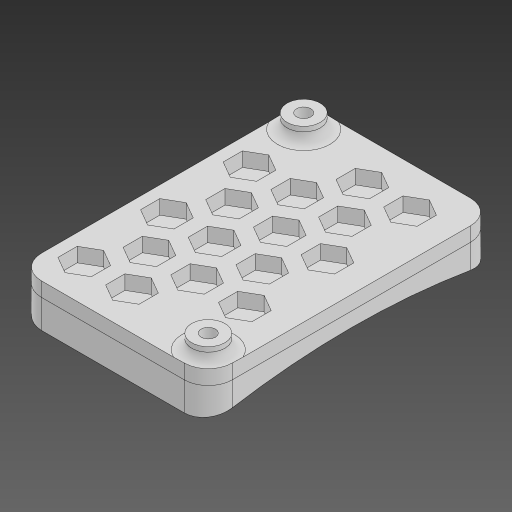
# Autodesk Inventor part: Base
Saved by Autodesk Inventor 2023.2 (Build 272271000, 271)
## iProperties
Created: 2023-04-07
Part Number: Base
Material: Generic
Document SubType Name: Modeling
Designer: jcgg2
Density: 1 g/cm^3
Appearance: Default
Mass: 14.6819 g
Surface Area: 110.672 cm^2
Volume: 14.6819 cm^3
Author: jcgg2
Autodesk Inventor part; units mm, degrees
ref_plane "YZ Plane" through (0, 0, 0) normal (1, 0, 0) x (0, 1, 0)
ref_plane "XZ Plane" through (0, 0, 0) normal (0, 1, 0) x (-1, 0, 0)
ref_plane "XY Plane" through (0, 0, 0) normal (0, 0, 1) x (1, 0, 0)
sketch "Sketch1" plane through (0, 0, 0) normal (0, 1, 0) x (-1, 0, 0)
  line L0 (-20, 30) -> (20, 30) construction
  line L1 (20, 30) -> (20, -30) construction
  line L2 (20, -30) -> (-20, -30) construction
  line L3 (-20, -30) -> (-20, 30) construction
  line L4 (-20, 30) -> (20, -30) construction
  line L5 (20, 30) -> (-20, -30) construction
  line L6 (-20, 30) -> (20, 30)
  line L7 (20, 30) -> (20, -30)
  line L8 (20, -30) -> (-20, -30)
  line L9 (-20, -30) -> (-20, 30)
  line L10 (-20, 30) -> (20, -30) construction
  line L11 (20, 30) -> (-20, -30) construction
  point P0 (0, 0)
  point P1 (-15, 25)
  point P2 (15, -25)
  dimension "d0" = 60
  dimension "d1" = 40
  dimension "d2" = 5
  dimension "d3" = 5
  dimension "d4" = 5
  dimension "d5" = 5
  constraints: 24 end point, 4 midpoint, 4 parallel, 2 horizontal, 2 perpendicular
  measures "d0" distance of L0.end L1.end
  measures "d1" distance of L1.end L2.end
  measures "d2" distance from line of L0 point (-15, 25)
  measures "d3" distance from line of L3 point (-15, 25)
  measures "d4" distance from line of L2 point (15, -25)
  measures "d5" distance from line of L1 point (15, -25)
extrude "Extrusion1" add sketch "Sketch1" along normal blind 3
hole "Hole1" at (15, 0, 25) at (-15, 0, -25) direction (0, 1, 0) diameter 3 depth 12 tip angle 118
sketch "Sketch2" plane through (0, 3, 0) normal (0, 1, 0) x (1, 0, 0)
  circle A0 centre (15, -25) radius 1.5 projected
  circle A1 centre (-15, 25) radius 1.5 projected
  line L0 (20, 30) -> (-20, 30) projected
  line L1 (-20, 30) -> (-20, -30) projected
  line L2 (-20, -30) -> (20, -30) projected
  line L3 (20, -30) -> (20, 30) projected
  circle A2 centre (15, -25) radius 3.5
  circle A3 centre (-15, 25) radius 3.5
  point P0 (0, 0)
  dimension "d15" = 2
  dimension "d16" = 2
  constraints: 2 centre point
  measures "d15" radial gap between concentric circles of A0 A2
  measures "d16" radial gap between concentric circles of A1 A3
extrude "Extrusion2" add sketch "Sketch2" along normal blind 3 contours A2 | A3
fillet "Fillet1" radius 2 2 edges at (11.5, 3, 25) (-18.5, 3, -25)
fillet "Fillet2" radius 5 4 edges at (20, 1.5, 30) (-20, 1.5, 30) (20, 1.5, -30) (-20, 1.5, -30)
sketch "Sketch3" plane through (20, 0, 25) normal (1, 0, 0) x (0, 0, -1)
  line L0 (-5, 3.0635) -> (-5, 0) projected
  line L1 (55, 0) -> (55, 3) projected
  line L2 (0, 0) -> (50, 0) projected
  line L3 (0, 0) -> (-5, 0) projected
  line L4 (55, 0) -> (50, 0) projected
  line L5 (0, 0) -> (-5, 0) projected
  line L6 (-5, 0) -> (55, 0)
  line L7 (55, 0) -> (55, -6)
  line L8 (55, -6) -> (-5, -6)
  line L9 (-5, -6) -> (-5, 0)
  line L10 (-5, 0) -> (55, 0)
  line L11 (55, 0) -> (55, -3)
  line L12 (55, -3) -> (-5, -3)
  line L13 (-5, -3) -> (-5, 0)
  arc A0 (55, -6) -> (-5, -6) centre (25, -154.5) ccw
  point P0 (25, 0)
  dimension "d21" = 6
  dimension "d22" = 3
  constraints: 16 end point, 4 parallel, 2 horizontal, 2 perpendicular, 2 point on circle, 1 centre point, 1 collinear, 1 midpoint, 1 tangent
  measures "d21" distance of L6.end L7.end
  measures "d22" distance of L10.end L11.end
extrude "Extrusion3" add sketch "Sketch3" against normal blind 40 separate body contours L2 L4 L7 L12 L9 L3 | L12 A0 L9 | L7 A0 L12
fillet "Fillet3" radius 5 4 edges at (20, -3, -30) (-20, -3, -30) (20, -3, 30) (-20, -3, 30)
sketch "Sketch4" plane through (20, 0, 25) normal (0, 1, 0) x (1, 0, 0)
  circle A0 centre (-5, 0) radius 1.5 projected
  circle A1 centre (-35, 50) radius 1.5 projected
  point P0 (-20, 25)
extrude "Extrusion4" cut sketch "Sketch4" against normal blind 40 bodies 2
sketch "Sketch5" plane through (0, 3, 0) normal (0, 1, 0) x (1, 0, 0)
  line L0 (-14, -17.9585) -> (-10.5, -19.9793)
  line L1 (-10.5, -19.9793) -> (-10.5, -24.0207)
  line L2 (-10.5, -24.0207) -> (-14, -26.0415)
  line L3 (-14, -26.0415) -> (-17.5, -24.0207)
  line L4 (-17.5, -24.0207) -> (-17.5, -19.9793)
  line L5 (-17.5, -19.9793) -> (-14, -17.9585)
  line L6 (-20, 22.7087) -> (-20, -25) projected
  line L7 (-15, -30) -> (12.7087, -30) projected
  line L8 (-14, -22) -> (-7.0718, -10) construction
  line L9 (-14, -22) -> (-7.0718, -22) construction
  line L10 (-4, -17.9585) -> (-0.5, -19.9793)
  line L11 (-0.5, -19.9793) -> (-0.5, -24.0207)
  line L12 (-0.5, -24.0207) -> (-4, -26.0415)
  line L13 (-4, -26.0415) -> (-7.5, -24.0207)
  line L14 (-7.5, -24.0207) -> (-7.5, -19.9793)
  line L15 (-7.5, -19.9793) -> (-4, -17.9585)
  line L16 (6, -17.9585) -> (9.5, -19.9793)
  line L17 (9.5, -19.9793) -> (9.5, -24.0207)
  line L18 (9.5, -24.0207) -> (6, -26.0415)
  line L19 (6, -26.0415) -> (2.5, -24.0207)
  line L20 (2.5, -24.0207) -> (2.5, -19.9793)
  line L21 (2.5, -19.9793) -> (6, -17.9585)
  line L22 (16, -17.9585) -> (19.5, -19.9793)
  line L23 (19.5, -19.9793) -> (19.5, -24.0207)
  line L24 (19.5, -24.0207) -> (16, -26.0415)
  line L25 (16, -26.0415) -> (12.5, -24.0207)
  line L26 (12.5, -24.0207) -> (12.5, -19.9793)
  line L27 (12.5, -19.9793) -> (16, -17.9585)
  line L28 (26, -17.9585) -> (29.5, -19.9793)
  line L29 (29.5, -19.9793) -> (29.5, -24.0207)
  line L30 (29.5, -24.0207) -> (26, -26.0415)
  line L31 (26, -26.0415) -> (22.5, -24.0207)
  line L32 (22.5, -24.0207) -> (22.5, -19.9793)
  line L33 (22.5, -19.9793) -> (26, -17.9585)
  line L34 (-9, -9.2983) -> (-5.5, -11.319)
  line L35 (-5.5, -11.319) -> (-5.5, -15.3605)
  line L36 (-5.5, -15.3605) -> (-9, -17.3812)
  line L37 (-9, -17.3812) -> (-12.5, -15.3605)
  line L38 (-12.5, -15.3605) -> (-12.5, -11.319)
  line L39 (-12.5, -11.319) -> (-9, -9.2983)
  line L40 (1, -9.2983) -> (4.5, -11.319)
  line L41 (4.5, -11.319) -> (4.5, -15.3605)
  line L42 (4.5, -15.3605) -> (1, -17.3812)
  line L43 (1, -17.3812) -> (-2.5, -15.3605)
  line L44 (-2.5, -15.3605) -> (-2.5, -11.319)
  line L45 (-2.5, -11.319) -> (1, -9.2983)
  line L46 (11, -9.2983) -> (14.5, -11.319)
  line L47 (14.5, -11.319) -> (14.5, -15.3605)
  line L48 (14.5, -15.3605) -> (11, -17.3812)
  line L49 (11, -17.3812) -> (7.5, -15.3605)
  line L50 (7.5, -15.3605) -> (7.5, -11.319)
  line L51 (7.5, -11.319) -> (11, -9.2983)
  line L52 (21, -9.2983) -> (24.5, -11.319)
  line L53 (24.5, -11.319) -> (24.5, -15.3605)
  line L54 (24.5, -15.3605) -> (21, -17.3812)
  line L55 (21, -17.3812) -> (17.5, -15.3605)
  line L56 (17.5, -15.3605) -> (17.5, -11.319)
  line L57 (17.5, -11.319) -> (21, -9.2983)
  line L58 (31, -9.2983) -> (34.5, -11.319)
  line L59 (34.5, -11.319) -> (34.5, -15.3605)
  line L60 (34.5, -15.3605) -> (31, -17.3812)
  line L61 (31, -17.3812) -> (27.5, -15.3605)
  line L62 (27.5, -15.3605) -> (27.5, -11.319)
  line L63 (27.5, -11.319) -> (31, -9.2983)
  line L64 (-4, -0.638) -> (-0.5, -2.6588)
  line L65 (-0.5, -2.6588) -> (-0.5, -6.7002)
  line L66 (-0.5, -6.7002) -> (-4, -8.7209)
  line L67 (-4, -8.7209) -> (-7.5, -6.7002)
  line L68 (-7.5, -6.7002) -> (-7.5, -2.6588)
  line L69 (-7.5, -2.6588) -> (-4, -0.638)
  line L70 (6, -0.638) -> (9.5, -2.6588)
  line L71 (9.5, -2.6588) -> (9.5, -6.7002)
  line L72 (9.5, -6.7002) -> (6, -8.7209)
  line L73 (6, -8.7209) -> (2.5, -6.7002)
  line L74 (2.5, -6.7002) -> (2.5, -2.6588)
  line L75 (2.5, -2.6588) -> (6, -0.638)
  line L76 (16, -0.638) -> (19.5, -2.6588)
  line L77 (19.5, -2.6588) -> (19.5, -6.7002)
  line L78 (19.5, -6.7002) -> (16, -8.7209)
  line L79 (16, -8.7209) -> (12.5, -6.7002)
  line L80 (12.5, -6.7002) -> (12.5, -2.6588)
  line L81 (12.5, -2.6588) -> (16, -0.638)
  line L82 (26, -0.638) -> (29.5, -2.6588)
  line L83 (29.5, -2.6588) -> (29.5, -6.7002)
  line L84 (29.5, -6.7002) -> (26, -8.7209)
  line L85 (26, -8.7209) -> (22.5, -6.7002)
  line L86 (22.5, -6.7002) -> (22.5, -2.6588)
  line L87 (22.5, -2.6588) -> (26, -0.638)
  line L88 (36, -0.638) -> (39.5, -2.6588)
  line L89 (39.5, -2.6588) -> (39.5, -6.7002)
  line L90 (39.5, -6.7002) -> (36, -8.7209)
  line L91 (36, -8.7209) -> (32.5, -6.7002)
  line L92 (32.5, -6.7002) -> (32.5, -2.6588)
  line L93 (32.5, -2.6588) -> (36, -0.638)
  line L94 (1, 8.0222) -> (4.5, 6.0015)
  line L95 (4.5, 6.0015) -> (4.5, 1.96)
  line L96 (4.5, 1.96) -> (1, -0.0607)
  line L97 (1, -0.0607) -> (-2.5, 1.96)
  line L98 (-2.5, 1.96) -> (-2.5, 6.0015)
  line L99 (-2.5, 6.0015) -> (1, 8.0222)
  line L100 (11, 8.0222) -> (14.5, 6.0015)
  line L101 (14.5, 6.0015) -> (14.5, 1.96)
  line L102 (14.5, 1.96) -> (11, -0.0607)
  line L103 (11, -0.0607) -> (7.5, 1.96)
  line L104 (7.5, 1.96) -> (7.5, 6.0015)
  line L105 (7.5, 6.0015) -> (11, 8.0222)
  line L106 (21, 8.0222) -> (24.5, 6.0015)
  line L107 (24.5, 6.0015) -> (24.5, 1.96)
  line L108 (24.5, 1.96) -> (21, -0.0607)
  line L109 (21, -0.0607) -> (17.5, 1.96)
  line L110 (17.5, 1.96) -> (17.5, 6.0015)
  line L111 (17.5, 6.0015) -> (21, 8.0222)
  line L112 (31, 8.0222) -> (34.5, 6.0015)
  line L113 (34.5, 6.0015) -> (34.5, 1.96)
  line L114 (34.5, 1.96) -> (31, -0.0607)
  line L115 (31, -0.0607) -> (27.5, 1.96)
  line L116 (27.5, 1.96) -> (27.5, 6.0015)
  line L117 (27.5, 6.0015) -> (31, 8.0222)
  line L118 (41, 8.0222) -> (44.5, 6.0015)
  line L119 (44.5, 6.0015) -> (44.5, 1.96)
  line L120 (44.5, 1.96) -> (41, -0.0607)
  line L121 (41, -0.0607) -> (37.5, 1.96)
  line L122 (37.5, 1.96) -> (37.5, 6.0015)
  line L123 (37.5, 6.0015) -> (41, 8.0222)
  line L124 (6, 16.6825) -> (9.5, 14.6617)
  line L125 (9.5, 14.6617) -> (9.5, 10.6203)
  line L126 (9.5, 10.6203) -> (6, 8.5996)
  line L127 (6, 8.5996) -> (2.5, 10.6203)
  line L128 (2.5, 10.6203) -> (2.5, 14.6617)
  line L129 (2.5, 14.6617) -> (6, 16.6825)
  line L130 (16, 16.6825) -> (19.5, 14.6617)
  line L131 (19.5, 14.6617) -> (19.5, 10.6203)
  line L132 (19.5, 10.6203) -> (16, 8.5996)
  line L133 (16, 8.5996) -> (12.5, 10.6203)
  line L134 (12.5, 10.6203) -> (12.5, 14.6617)
  line L135 (12.5, 14.6617) -> (16, 16.6825)
  line L136 (26, 16.6825) -> (29.5, 14.6617)
  line L137 (29.5, 14.6617) -> (29.5, 10.6203)
  line L138 (29.5, 10.6203) -> (26, 8.5996)
  line L139 (26, 8.5996) -> (22.5, 10.6203)
  line L140 (22.5, 10.6203) -> (22.5, 14.6617)
  line L141 (22.5, 14.6617) -> (26, 16.6825)
  line L142 (36, 16.6825) -> (39.5, 14.6617)
  line L143 (39.5, 14.6617) -> (39.5, 10.6203)
  line L144 (39.5, 10.6203) -> (36, 8.5996)
  line L145 (36, 8.5996) -> (32.5, 10.6203)
  line L146 (32.5, 10.6203) -> (32.5, 14.6617)
  line L147 (32.5, 14.6617) -> (36, 16.6825)
  line L148 (46, 16.6825) -> (49.5, 14.6617)
  line L149 (49.5, 14.6617) -> (49.5, 10.6203)
  line L150 (49.5, 10.6203) -> (46, 8.5996)
  line L151 (46, 8.5996) -> (42.5, 10.6203)
  line L152 (42.5, 10.6203) -> (42.5, 14.6617)
  line L153 (42.5, 14.6617) -> (46, 16.6825)
  line L154 (11, 25.3427) -> (14.5, 23.322)
  line L155 (14.5, 23.322) -> (14.5, 19.2805)
  line L156 (14.5, 19.2805) -> (11, 17.2598)
  line L157 (11, 17.2598) -> (7.5, 19.2805)
  line L158 (7.5, 19.2805) -> (7.5, 23.322)
  line L159 (7.5, 23.322) -> (11, 25.3427)
  line L160 (21, 25.3427) -> (24.5, 23.322)
  line L161 (24.5, 23.322) -> (24.5, 19.2805)
  line L162 (24.5, 19.2805) -> (21, 17.2598)
  line L163 (21, 17.2598) -> (17.5, 19.2805)
  line L164 (17.5, 19.2805) -> (17.5, 23.322)
  line L165 (17.5, 23.322) -> (21, 25.3427)
  line L166 (31, 25.3427) -> (34.5, 23.322)
  line L167 (34.5, 23.322) -> (34.5, 19.2805)
  line L168 (34.5, 19.2805) -> (31, 17.2598)
  line L169 (31, 17.2598) -> (27.5, 19.2805)
  line L170 (27.5, 19.2805) -> (27.5, 23.322)
  line L171 (27.5, 23.322) -> (31, 25.3427)
  line L172 (41, 25.3427) -> (44.5, 23.322)
  line L173 (44.5, 23.322) -> (44.5, 19.2805)
  line L174 (44.5, 19.2805) -> (41, 17.2598)
  line L175 (41, 17.2598) -> (37.5, 19.2805)
  line L176 (37.5, 19.2805) -> (37.5, 23.322)
  line L177 (37.5, 23.322) -> (41, 25.3427)
  line L178 (51, 25.3427) -> (54.5, 23.322)
  line L179 (54.5, 23.322) -> (54.5, 19.2805)
  line L180 (54.5, 19.2805) -> (51, 17.2598)
  line L181 (51, 17.2598) -> (47.5, 19.2805)
  line L182 (47.5, 19.2805) -> (47.5, 23.322)
  line L183 (47.5, 23.322) -> (51, 25.3427)
  line L184 (16, 34.003) -> (19.5, 31.9823)
  line L185 (19.5, 31.9823) -> (19.5, 27.9408)
  line L186 (19.5, 27.9408) -> (16, 25.9201)
  line L187 (16, 25.9201) -> (12.5, 27.9408)
  line L188 (12.5, 27.9408) -> (12.5, 31.9823)
  line L189 (12.5, 31.9823) -> (16, 34.003)
  line L190 (26, 34.003) -> (29.5, 31.9823)
  line L191 (29.5, 31.9823) -> (29.5, 27.9408)
  line L192 (29.5, 27.9408) -> (26, 25.9201)
  line L193 (26, 25.9201) -> (22.5, 27.9408)
  line L194 (22.5, 27.9408) -> (22.5, 31.9823)
  line L195 (22.5, 31.9823) -> (26, 34.003)
  line L196 (36, 34.003) -> (39.5, 31.9823)
  line L197 (39.5, 31.9823) -> (39.5, 27.9408)
  line L198 (39.5, 27.9408) -> (36, 25.9201)
  line L199 (36, 25.9201) -> (32.5, 27.9408)
  line L200 (32.5, 27.9408) -> (32.5, 31.9823)
  line L201 (32.5, 31.9823) -> (36, 34.003)
  line L202 (46, 34.003) -> (49.5, 31.9823)
  line L203 (49.5, 31.9823) -> (49.5, 27.9408)
  line L204 (49.5, 27.9408) -> (46, 25.9201)
  line L205 (46, 25.9201) -> (42.5, 27.9408)
  line L206 (42.5, 27.9408) -> (42.5, 31.9823)
  line L207 (42.5, 31.9823) -> (46, 34.003)
  line L208 (56, 34.003) -> (59.5, 31.9823)
  line L209 (59.5, 31.9823) -> (59.5, 27.9408)
  line L210 (59.5, 27.9408) -> (56, 25.9201)
  line L211 (56, 25.9201) -> (52.5, 27.9408)
  line L212 (52.5, 27.9408) -> (52.5, 31.9823)
  line L213 (52.5, 31.9823) -> (56, 34.003)
  line L214 (-20.5, -24.0207) -> (-24, -26.0415)
  line L215 (-24, -26.0415) -> (-27.5, -24.0207)
  line L216 (-24, -17.9585) -> (-20.5, -19.9793)
  line L217 (-20.5, -19.9793) -> (-20.5, -24.0207)
  line L218 (-27.5, -24.0207) -> (-27.5, -19.9793)
  line L219 (-27.5, -19.9793) -> (-24, -17.9585)
  line L220 (-30.5, -24.0207) -> (-34, -26.0415)
  line L221 (-34, -26.0415) -> (-37.5, -24.0207)
  line L222 (-34, -17.9585) -> (-30.5, -19.9793)
  line L223 (-30.5, -19.9793) -> (-30.5, -24.0207)
  line L224 (-37.5, -24.0207) -> (-37.5, -19.9793)
  line L225 (-37.5, -19.9793) -> (-34, -17.9585)
  line L226 (-40.5, -24.0207) -> (-44, -26.0415)
  line L227 (-44, -26.0415) -> (-47.5, -24.0207)
  line L228 (-44, -17.9585) -> (-40.5, -19.9793)
  line L229 (-40.5, -19.9793) -> (-40.5, -24.0207)
  line L230 (-47.5, -24.0207) -> (-47.5, -19.9793)
  line L231 (-47.5, -19.9793) -> (-44, -17.9585)
  line L232 (-50.5, -24.0207) -> (-54, -26.0415)
  line L233 (-54, -26.0415) -> (-57.5, -24.0207)
  line L234 (-54, -17.9585) -> (-50.5, -19.9793)
  line L235 (-50.5, -19.9793) -> (-50.5, -24.0207)
  line L236 (-57.5, -24.0207) -> (-57.5, -19.9793)
  line L237 (-57.5, -19.9793) -> (-54, -17.9585)
  line L238 (-5.5, -15.3605) -> (-9, -17.3812)
  line L239 (-9, -17.3812) -> (-12.5, -15.3605)
  line L240 (-9, -9.2983) -> (-5.5, -11.319)
  line L241 (-5.5, -11.319) -> (-5.5, -15.3605)
  line L242 (-12.5, -15.3605) -> (-12.5, -11.319)
  line L243 (-12.5, -11.319) -> (-9, -9.2983)
  line L244 (-15.5, -15.3605) -> (-19, -17.3812)
  line L245 (-19, -17.3812) -> (-22.5, -15.3605)
  line L246 (-19, -9.2983) -> (-15.5, -11.319)
  line L247 (-15.5, -11.319) -> (-15.5, -15.3605)
  line L248 (-22.5, -15.3605) -> (-22.5, -11.319)
  line L249 (-22.5, -11.319) -> (-19, -9.2983)
  line L250 (-25.5, -15.3605) -> (-29, -17.3812)
  line L251 (-29, -17.3812) -> (-32.5, -15.3605)
  line L252 (-29, -9.2983) -> (-25.5, -11.319)
  line L253 (-25.5, -11.319) -> (-25.5, -15.3605)
  line L254 (-32.5, -15.3605) -> (-32.5, -11.319)
  line L255 (-32.5, -11.319) -> (-29, -9.2983)
  line L256 (-35.5, -15.3605) -> (-39, -17.3812)
  line L257 (-39, -17.3812) -> (-42.5, -15.3605)
  line L258 (-39, -9.2983) -> (-35.5, -11.319)
  line L259 (-35.5, -11.319) -> (-35.5, -15.3605)
  line L260 (-42.5, -15.3605) -> (-42.5, -11.319)
  line L261 (-42.5, -11.319) -> (-39, -9.2983)
  line L262 (-45.5, -15.3605) -> (-49, -17.3812)
  line L263 (-49, -17.3812) -> (-52.5, -15.3605)
  line L264 (-49, -9.2983) -> (-45.5, -11.319)
  line L265 (-45.5, -11.319) -> (-45.5, -15.3605)
  line L266 (-52.5, -15.3605) -> (-52.5, -11.319)
  line L267 (-52.5, -11.319) -> (-49, -9.2983)
  line L268 (-0.5, -6.7002) -> (-4, -8.7209)
  line L269 (-4, -8.7209) -> (-7.5, -6.7002)
  line L270 (-4, -0.638) -> (-0.5, -2.6588)
  line L271 (-0.5, -2.6588) -> (-0.5, -6.7002)
  line L272 (-7.5, -6.7002) -> (-7.5, -2.6588)
  line L273 (-7.5, -2.6588) -> (-4, -0.638)
  line L274 (-10.5, -6.7002) -> (-14, -8.7209)
  line L275 (-14, -8.7209) -> (-17.5, -6.7002)
  line L276 (-14, -0.638) -> (-10.5, -2.6588)
  line L277 (-10.5, -2.6588) -> (-10.5, -6.7002)
  line L278 (-17.5, -6.7002) -> (-17.5, -2.6588)
  line L279 (-17.5, -2.6588) -> (-14, -0.638)
  line L280 (-20.5, -6.7002) -> (-24, -8.7209)
  line L281 (-24, -8.7209) -> (-27.5, -6.7002)
  line L282 (-24, -0.638) -> (-20.5, -2.6588)
  line L283 (-20.5, -2.6588) -> (-20.5, -6.7002)
  line L284 (-27.5, -6.7002) -> (-27.5, -2.6588)
  line L285 (-27.5, -2.6588) -> (-24, -0.638)
  line L286 (-30.5, -6.7002) -> (-34, -8.7209)
  line L287 (-34, -8.7209) -> (-37.5, -6.7002)
  line L288 (-34, -0.638) -> (-30.5, -2.6588)
  line L289 (-30.5, -2.6588) -> (-30.5, -6.7002)
  line L290 (-37.5, -6.7002) -> (-37.5, -2.6588)
  line L291 (-37.5, -2.6588) -> (-34, -0.638)
  line L292 (-40.5, -6.7002) -> (-44, -8.7209)
  line L293 (-44, -8.7209) -> (-47.5, -6.7002)
  line L294 (-44, -0.638) -> (-40.5, -2.6588)
  line L295 (-40.5, -2.6588) -> (-40.5, -6.7002)
  line L296 (-47.5, -6.7002) -> (-47.5, -2.6588)
  line L297 (-47.5, -2.6588) -> (-44, -0.638)
  line L298 (4.5, 1.96) -> (1, -0.0607)
  line L299 (1, -0.0607) -> (-2.5, 1.96)
  line L300 (1, 8.0222) -> (4.5, 6.0015)
  line L301 (4.5, 6.0015) -> (4.5, 1.96)
  line L302 (-2.5, 1.96) -> (-2.5, 6.0015)
  line L303 (-2.5, 6.0015) -> (1, 8.0222)
  line L304 (-5.5, 1.96) -> (-9, -0.0607)
  line L305 (-9, -0.0607) -> (-12.5, 1.96)
  line L306 (-9, 8.0222) -> (-5.5, 6.0015)
  line L307 (-5.5, 6.0015) -> (-5.5, 1.96)
  line L308 (-12.5, 1.96) -> (-12.5, 6.0015)
  line L309 (-12.5, 6.0015) -> (-9, 8.0222)
  line L310 (-15.5, 1.96) -> (-19, -0.0607)
  line L311 (-19, -0.0607) -> (-22.5, 1.96)
  line L312 (-19, 8.0222) -> (-15.5, 6.0015)
  line L313 (-15.5, 6.0015) -> (-15.5, 1.96)
  line L314 (-22.5, 1.96) -> (-22.5, 6.0015)
  line L315 (-22.5, 6.0015) -> (-19, 8.0222)
  line L316 (-25.5, 1.96) -> (-29, -0.0607)
  line L317 (-29, -0.0607) -> (-32.5, 1.96)
  line L318 (-29, 8.0222) -> (-25.5, 6.0015)
  line L319 (-25.5, 6.0015) -> (-25.5, 1.96)
  line L320 (-32.5, 1.96) -> (-32.5, 6.0015)
  line L321 (-32.5, 6.0015) -> (-29, 8.0222)
  line L322 (-35.5, 1.96) -> (-39, -0.0607)
  line L323 (-39, -0.0607) -> (-42.5, 1.96)
  line L324 (-39, 8.0222) -> (-35.5, 6.0015)
  line L325 (-35.5, 6.0015) -> (-35.5, 1.96)
  line L326 (-42.5, 1.96) -> (-42.5, 6.0015)
  line L327 (-42.5, 6.0015) -> (-39, 8.0222)
  line L328 (9.5, 10.6203) -> (6, 8.5996)
  line L329 (6, 8.5996) -> (2.5, 10.6203)
  line L330 (6, 16.6825) -> (9.5, 14.6617)
  line L331 (9.5, 14.6617) -> (9.5, 10.6203)
  line L332 (2.5, 10.6203) -> (2.5, 14.6617)
  line L333 (2.5, 14.6617) -> (6, 16.6825)
  line L334 (-0.5, 10.6203) -> (-4, 8.5996)
  line L335 (-4, 8.5996) -> (-7.5, 10.6203)
  line L336 (-4, 16.6825) -> (-0.5, 14.6617)
  line L337 (-0.5, 14.6617) -> (-0.5, 10.6203)
  line L338 (-7.5, 10.6203) -> (-7.5, 14.6617)
  line L339 (-7.5, 14.6617) -> (-4, 16.6825)
  line L340 (-10.5, 10.6203) -> (-14, 8.5996)
  line L341 (-14, 8.5996) -> (-17.5, 10.6203)
  line L342 (-14, 16.6825) -> (-10.5, 14.6617)
  line L343 (-10.5, 14.6617) -> (-10.5, 10.6203)
  line L344 (-17.5, 10.6203) -> (-17.5, 14.6617)
  line L345 (-17.5, 14.6617) -> (-14, 16.6825)
  line L346 (-20.5, 10.6203) -> (-24, 8.5996)
  line L347 (-24, 8.5996) -> (-27.5, 10.6203)
  line L348 (-24, 16.6825) -> (-20.5, 14.6617)
  line L349 (-20.5, 14.6617) -> (-20.5, 10.6203)
  line L350 (-27.5, 10.6203) -> (-27.5, 14.6617)
  line L351 (-27.5, 14.6617) -> (-24, 16.6825)
  line L352 (-30.5, 10.6203) -> (-34, 8.5996)
  line L353 (-34, 8.5996) -> (-37.5, 10.6203)
  line L354 (-34, 16.6825) -> (-30.5, 14.6617)
  line L355 (-30.5, 14.6617) -> (-30.5, 10.6203)
  line L356 (-37.5, 10.6203) -> (-37.5, 14.6617)
  line L357 (-37.5, 14.6617) -> (-34, 16.6825)
  line L358 (14.5, 19.2805) -> (11, 17.2598)
  line L359 (11, 17.2598) -> (7.5, 19.2805)
  line L360 (11, 25.3427) -> (14.5, 23.322)
  line L361 (14.5, 23.322) -> (14.5, 19.2805)
  line L362 (7.5, 19.2805) -> (7.5, 23.322)
  line L363 (7.5, 23.322) -> (11, 25.3427)
  line L364 (4.5, 19.2805) -> (1, 17.2598)
  line L365 (1, 17.2598) -> (-2.5, 19.2805)
  line L366 (1, 25.3427) -> (4.5, 23.322)
  line L367 (4.5, 23.322) -> (4.5, 19.2805)
  line L368 (-2.5, 19.2805) -> (-2.5, 23.322)
  line L369 (-2.5, 23.322) -> (1, 25.3427)
  line L370 (-5.5, 19.2805) -> (-9, 17.2598)
  line L371 (-9, 17.2598) -> (-12.5, 19.2805)
  line L372 (-9, 25.3427) -> (-5.5, 23.322)
  line L373 (-5.5, 23.322) -> (-5.5, 19.2805)
  line L374 (-12.5, 19.2805) -> (-12.5, 23.322)
  line L375 (-12.5, 23.322) -> (-9, 25.3427)
  line L376 (-15.5, 19.2805) -> (-19, 17.2598)
  line L377 (-19, 17.2598) -> (-22.5, 19.2805)
  line L378 (-19, 25.3427) -> (-15.5, 23.322)
  line L379 (-15.5, 23.322) -> (-15.5, 19.2805)
  line L380 (-22.5, 19.2805) -> (-22.5, 23.322)
  line L381 (-22.5, 23.322) -> (-19, 25.3427)
  line L382 (-25.5, 19.2805) -> (-29, 17.2598)
  line L383 (-29, 17.2598) -> (-32.5, 19.2805)
  line L384 (-29, 25.3427) -> (-25.5, 23.322)
  line L385 (-25.5, 23.322) -> (-25.5, 19.2805)
  line L386 (-32.5, 19.2805) -> (-32.5, 23.322)
  line L387 (-32.5, 23.322) -> (-29, 25.3427)
  line L388 (19.5, 27.9408) -> (16, 25.9201)
  line L389 (16, 25.9201) -> (12.5, 27.9408)
  line L390 (16, 34.003) -> (19.5, 31.9823)
  line L391 (19.5, 31.9823) -> (19.5, 27.9408)
  line L392 (12.5, 27.9408) -> (12.5, 31.9823)
  line L393 (12.5, 31.9823) -> (16, 34.003)
  line L394 (9.5, 27.9408) -> (6, 25.9201)
  line L395 (6, 25.9201) -> (2.5, 27.9408)
  line L396 (6, 34.003) -> (9.5, 31.9823)
  line L397 (9.5, 31.9823) -> (9.5, 27.9408)
  line L398 (2.5, 27.9408) -> (2.5, 31.9823)
  line L399 (2.5, 31.9823) -> (6, 34.003)
  line L400 (-0.5, 27.9408) -> (-4, 25.9201)
  line L401 (-4, 25.9201) -> (-7.5, 27.9408)
  line L402 (-4, 34.003) -> (-0.5, 31.9823)
  line L403 (-0.5, 31.9823) -> (-0.5, 27.9408)
  line L404 (-7.5, 27.9408) -> (-7.5, 31.9823)
  line L405 (-7.5, 31.9823) -> (-4, 34.003)
  line L406 (-10.5, 27.9408) -> (-14, 25.9201)
  line L407 (-14, 25.9201) -> (-17.5, 27.9408)
  line L408 (-14, 34.003) -> (-10.5, 31.9823)
  line L409 (-10.5, 31.9823) -> (-10.5, 27.9408)
  line L410 (-17.5, 27.9408) -> (-17.5, 31.9823)
  line L411 (-17.5, 31.9823) -> (-14, 34.003)
  line L412 (-20.5, 27.9408) -> (-24, 25.9201)
  line L413 (-24, 25.9201) -> (-27.5, 27.9408)
  line L414 (-24, 34.003) -> (-20.5, 31.9823)
  line L415 (-20.5, 31.9823) -> (-20.5, 27.9408)
  line L416 (-27.5, 27.9408) -> (-27.5, 31.9823)
  line L417 (-27.5, 31.9823) -> (-24, 34.003)
  point P0 (0, 0)
  point P1 (-17.5, -22)
  point P2 (-10.5, -22)
  point P3 (-4, -22)
  point P4 (-0.5, -22)
  point P5 (-7.5, -22)
  point P6 (6, -22)
  point P7 (9.5, -22)
  point P8 (2.5, -22)
  point P9 (16, -22)
  point P10 (19.5, -22)
  point P11 (12.5, -22)
  point P12 (26, -22)
  point P13 (29.5, -22)
  point P14 (22.5, -22)
  point P15 (-9, -13.3397)
  point P16 (-5.5, -13.3397)
  point P17 (-12.5, -13.3397)
  point P18 (1, -13.3397)
  point P19 (4.5, -13.3397)
  point P20 (-2.5, -13.3397)
  point P21 (11, -13.3397)
  point P22 (14.5, -13.3397)
  point P23 (7.5, -13.3397)
  point P24 (21, -13.3397)
  point P25 (24.5, -13.3397)
  point P26 (17.5, -13.3397)
  point P27 (31, -13.3397)
  point P28 (34.5, -13.3397)
  point P29 (27.5, -13.3397)
  point P30 (-4, -4.6795)
  point P31 (-0.5, -4.6795)
  point P32 (-7.5, -4.6795)
  point P33 (6, -4.6795)
  point P34 (9.5, -4.6795)
  point P35 (2.5, -4.6795)
  point P36 (16, -4.6795)
  point P37 (19.5, -4.6795)
  point P38 (12.5, -4.6795)
  point P39 (26, -4.6795)
  point P40 (29.5, -4.6795)
  point P41 (22.5, -4.6795)
  point P42 (36, -4.6795)
  point P43 (39.5, -4.6795)
  point P44 (32.5, -4.6795)
  point P45 (1, 3.9808)
  point P46 (4.5, 3.9808)
  point P47 (-2.5, 3.9808)
  point P48 (11, 3.9808)
  point P49 (14.5, 3.9808)
  point P50 (7.5, 3.9808)
  point P51 (21, 3.9808)
  point P52 (24.5, 3.9808)
  point P53 (17.5, 3.9808)
  point P54 (31, 3.9808)
  point P55 (34.5, 3.9808)
  point P56 (27.5, 3.9808)
  point P57 (41, 3.9808)
  point P58 (44.5, 3.9808)
  point P59 (37.5, 3.9808)
  point P60 (6, 12.641)
  point P61 (9.5, 12.641)
  point P62 (2.5, 12.641)
  point P63 (16, 12.641)
  point P64 (19.5, 12.641)
  point P65 (12.5, 12.641)
  point P66 (26, 12.641)
  point P67 (29.5, 12.641)
  point P68 (22.5, 12.641)
  point P69 (36, 12.641)
  point P70 (39.5, 12.641)
  point P71 (32.5, 12.641)
  point P72 (46, 12.641)
  point P73 (49.5, 12.641)
  point P74 (42.5, 12.641)
  point P75 (11, 21.3013)
  point P76 (14.5, 21.3013)
  point P77 (7.5, 21.3013)
  point P78 (21, 21.3013)
  point P79 (24.5, 21.3013)
  point P80 (17.5, 21.3013)
  point P81 (31, 21.3013)
  point P82 (34.5, 21.3013)
  point P83 (27.5, 21.3013)
  point P84 (41, 21.3013)
  point P85 (44.5, 21.3013)
  point P86 (37.5, 21.3013)
  point P87 (51, 21.3013)
  point P88 (54.5, 21.3013)
  point P89 (47.5, 21.3013)
  point P90 (16, 29.9615)
  point P91 (19.5, 29.9615)
  point P92 (12.5, 29.9615)
  point P93 (26, 29.9615)
  point P94 (29.5, 29.9615)
  point P95 (22.5, 29.9615)
  point P96 (36, 29.9615)
  point P97 (39.5, 29.9615)
  point P98 (32.5, 29.9615)
  point P99 (46, 29.9615)
  point P100 (49.5, 29.9615)
  point P101 (42.5, 29.9615)
  point P102 (56, 29.9615)
  point P103 (59.5, 29.9615)
  point P104 (52.5, 29.9615)
  point P105 (-24, -22)
  point P106 (-20.5, -22)
  point P107 (-27.5, -22)
  point P108 (-34, -22)
  point P109 (-30.5, -22)
  point P110 (-37.5, -22)
  point P111 (-44, -22)
  point P112 (-40.5, -22)
  point P113 (-47.5, -22)
  point P114 (-54, -22)
  point P115 (-50.5, -22)
  point P116 (-57.5, -22)
  point P117 (-9, -13.3397)
  point P118 (-5.5, -13.3397)
  point P119 (-12.5, -13.3397)
  point P120 (-19, -13.3397)
  point P121 (-15.5, -13.3397)
  point P122 (-22.5, -13.3397)
  point P123 (-29, -13.3397)
  point P124 (-25.5, -13.3397)
  point P125 (-32.5, -13.3397)
  point P126 (-39, -13.3397)
  point P127 (-35.5, -13.3397)
  point P128 (-42.5, -13.3397)
  point P129 (-49, -13.3397)
  point P130 (-45.5, -13.3397)
  point P131 (-52.5, -13.3397)
  point P132 (-4, -4.6795)
  point P133 (-0.5, -4.6795)
  point P134 (-7.5, -4.6795)
  point P135 (-14, -4.6795)
  point P136 (-10.5, -4.6795)
  point P137 (-17.5, -4.6795)
  point P138 (-24, -4.6795)
  point P139 (-20.5, -4.6795)
  point P140 (-27.5, -4.6795)
  point P141 (-34, -4.6795)
  point P142 (-30.5, -4.6795)
  point P143 (-37.5, -4.6795)
  point P144 (-44, -4.6795)
  point P145 (-40.5, -4.6795)
  point P146 (-47.5, -4.6795)
  point P147 (1, 3.9808)
  point P148 (4.5, 3.9808)
  point P149 (-2.5, 3.9808)
  point P150 (-9, 3.9808)
  point P151 (-5.5, 3.9808)
  point P152 (-12.5, 3.9808)
  point P153 (-19, 3.9808)
  point P154 (-15.5, 3.9808)
  point P155 (-22.5, 3.9808)
  point P156 (-29, 3.9808)
  point P157 (-25.5, 3.9808)
  point P158 (-32.5, 3.9808)
  point P159 (-39, 3.9808)
  point P160 (-35.5, 3.9808)
  point P161 (-42.5, 3.9808)
  point P162 (6, 12.641)
  point P163 (9.5, 12.641)
  point P164 (2.5, 12.641)
  point P165 (-4, 12.641)
  point P166 (-0.5, 12.641)
  point P167 (-7.5, 12.641)
  point P168 (-14, 12.641)
  point P169 (-10.5, 12.641)
  point P170 (-17.5, 12.641)
  point P171 (-24, 12.641)
  point P172 (-20.5, 12.641)
  point P173 (-27.5, 12.641)
  point P174 (-34, 12.641)
  point P175 (-30.5, 12.641)
  point P176 (-37.5, 12.641)
  point P177 (11, 21.3013)
  point P178 (14.5, 21.3013)
  point P179 (7.5, 21.3013)
  point P180 (1, 21.3013)
  point P181 (4.5, 21.3013)
  point P182 (-2.5, 21.3013)
  point P183 (-9, 21.3013)
  point P184 (-5.5, 21.3013)
  point P185 (-12.5, 21.3013)
  point P186 (-19, 21.3013)
  point P187 (-15.5, 21.3013)
  point P188 (-22.5, 21.3013)
  point P189 (-29, 21.3013)
  point P190 (-25.5, 21.3013)
  point P191 (-32.5, 21.3013)
  point P192 (16, 29.9615)
  point P193 (19.5, 29.9615)
  point P194 (12.5, 29.9615)
  point P195 (6, 29.9615)
  point P196 (9.5, 29.9615)
  point P197 (2.5, 29.9615)
  point P198 (-4, 29.9615)
  point P199 (-0.5, 29.9615)
  dimension "d28" = 7
  dimension "d29" = 6
  dimension "d30" = 8
  dimension "d33" = 10
  dimension "d36" = 10
  dimension "d41" = 10
  dimension "d44" = 10
  constraints: 832 end point, 3 horizontal, 2 midpoint, 1 perpendicular, 1 vertical, 1035 other
  measures "d28" distance of point (-17.5, -22) point (-10.5, -22)
  measures "d29" distance from line of L6 L8.start
  measures "d30" distance from line of L7 L8.start
  measures "d33" distance of L8.start point (-4, -22)
  measures "d36" distance of L8.start point (-9, -13.34)
  measures "d41" distance of L8.start point (-24, -22)
  measures "d44" distance of L8.start point (-9, -13.34)
extrude "Extrusion5" cut sketch "Sketch5" against normal blind 3 contours L0 L1 L2 L3 L4 L5 | L10 L11 L12 L13 L14 L15 | L34 L35 L36 L37 L38 L39 | L40 L41 L42 L43 L44 L45 | L46 L47 L48 L49 L50 L51 | L64 L65 L66 L67 L68 L69 | L70 L71 L72 L73 L74 L75 | L94 L95 L96 L97 L98 L99 | L100 L101 L102 L103 L104 L105 | L124 L125 L126 L127 L128 L129 | L154 L155 L156 L157 L158 L159 | L274 L275 L278 L279 L276 L277 | L304 L305 L308 L309 L306 L307 | L334 L335 L338 L339 L336 L337 | L340 L341 L344 L345 L342 L343 | L364 L365 L368 L369 L366 L367 bodies 1
